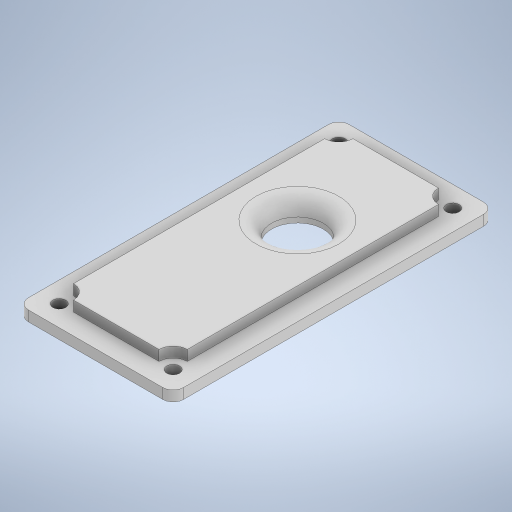
# Autodesk Inventor part: 커튼 서보 커버
Saved by Autodesk Inventor 2023.1 (Build 271208000, 208)
## iProperties
Created: 2022-09-03
Part Number: 커튼 서보 커버
Material: 일반
Document SubType Name: Modeling
Designer: fly01
Density: 1 g/cm^3
Appearance: 기본값
Author: fly01
Autodesk Inventor part; units mm, degrees
ref_plane "YZ Plane" through (0, 0, 0) normal (1, 0, 0) x (0, 1, 0)
ref_plane "XZ Plane" through (0, 0, 0) normal (0, 1, 0) x (-1, 0, 0)
ref_plane "XY Plane" through (0, 0, 0) normal (0, 0, 1) x (1, 0, 0)
sketch "스케치1" plane through (0, 0, 0) normal (0, 1, 0) x (-1, 0, 0)
  line L0 (11, 27) -> (-11, 27)
  line L1 (-11, 27) -> (-11, -27)
  line L2 (-11, -27) -> (11, -27)
  line L3 (11, -27) -> (11, 27)
  line L4 (11, 27) -> (-11, -27) construction
  line L5 (-11, 27) -> (11, -27) construction
  line L6 (15, 31) -> (-15, 31)
  line L7 (-15, 31) -> (-15, -31)
  line L8 (-15, -31) -> (15, -31)
  line L9 (15, -31) -> (15, 31)
  circle A0 centre (11, 27) radius 1.25
  line L10 (0, 0) -> (0, -5.338)
  line L11 (0, 0) -> (0.8274, 0)
  line L12 (0, 0) -> (4.4604, 0)
  circle A1 centre (11, 27) radius 2.75
  circle A2 centre (11, -27) radius 1.25
  circle A3 centre (11, -27) radius 2.75
  circle A4 centre (-11, 27) radius 1.25
  circle A5 centre (-11, 27) radius 2.75
  circle A6 centre (-11, -27) radius 1.25
  circle A7 centre (-11, -27) radius 2.75
  point P0 (-11, -24.25)
  point P1 (-8.25, -27)
  point P2 (8.25, -27)
  point P3 (11, -24.25)
  point P4 (11, 24.25)
  point P5 (8.25, 27)
  point P6 (-8.25, 27)
  point P7 (-11, 24.25)
  dimension "d0" = 22
  dimension "d1" = 54
  dimension "d2" = 4
  dimension "d3" = 2.5
  dimension "d4" = 5.5
  constraints: 26 end point, 8 centre point, 8 coincident, 6 symmetric about line, 4 parallel, 2 horizontal, 2 midpoint, 2 perpendicular, 1 vertical, 9 other
  measures "d0" distance of L2.end L1.end
  measures "d1" distance of L1.end L0.end
  measures "d2" distance between parallel lines of L3 L9
  measures "d3" diameter of A0
  measures "d4" diameter of A1
extrude "돌출1" add sketch "스케치1" against normal blind 2 contours A5 L1 A4 L0 | L0 A4 L1 A5 | L0 A1 L3 A3 L2 A7 L1 A5 | A1 L3 A0 L0 | L0 A0 L3 A1 | A7 L2 A6 L1 | L1 A6 L2 A7 | A3 L2 A2 L3 | L3 A2 L2 A3 | L9 L8 L7 L6
extrude "돌출2" add sketch "스케치1" along normal blind 2 contours L0 A1 L3 A3 L2 A7 L1 A5
fillet "모깎기1" radius 2 4 edges at (15, -1, -31) (-15, -1, -31) (15, -1, 31) (-15, -1, 31)
sketch "스케치2" plane through (0, 2, 0) normal (0, 1, 0) x (1, 0, 0)
  circle A0 centre (0, 8) radius 5
  line L0 (13, 31) -> (-13, 31) projected
  point P0 (0, 0)
  dimension "d10" = 23
  dimension "d11" = 10
  constraints: 1 centre point
  measures "d10" distance from line of L0 A0.centre
  measures "d11" diameter of A0
extrude "돌출3" cut sketch "스케치2" against normal blind 4
fillet "모깎기2" radius 3 1 edges at (-5, 2, -8)
